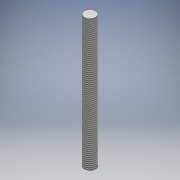
# Autodesk Inventor part: Pieza de unión
Saved by Autodesk Inventor 2018 (Build 220112000, 112)
## iProperties
Created: 2019-11-25
Part Number: Pieza de unión
Material: Genérico
Document SubType Name: Modeling
Designer: juanm
Density: 1 g/cm^3
Appearance: Valor por defecto
Author: juanm
Autodesk Inventor part; units mm, degrees
ref_plane "YZ Plane" through (0, 0, 0) normal (1, 0, 0) x (0, 1, 0)
ref_plane "XZ Plane" through (0, 0, 0) normal (0, 1, 0) x (-1, 0, 0)
ref_plane "XY Plane" through (0, 0, 0) normal (0, 0, 1) x (1, 0, 0)
sketch "Boceto1" plane through (0, 0, 0) normal (0, 0, 1) x (1, 0, 0)
  circle A0 centre (-17.2121, 9.1059) radius 6.35
  point P0 (0, 0)
  dimension "d0" = 12.7
  constraints: 1 centre point
  measures "d0" diameter of A0
extrude "Extrusión1" add sketch "Boceto1" along normal blind 150
thread "Rosca1" size "M14x2" class "6g" standard "ANSI Metric M Profile" full length
